nixal_reprap4040_rampsBracket (Autodesk Fusion 360 design; units mm, degrees)
Autodesk Fusion 360 part; units mm, degrees
sketch "Sketch1" plane through (0, 0, 0) normal (0, 1, 0) x (1, 0, 0)
  line L0 (0, 0) -> (135, 0)
  line L1 (135, 0) -> (135, 60)
  line L2 (135, 60) -> (0, 60)
  line L3 (0, 60) -> (0, 0)
  circle A0 centre (30, 10) radius 4
  circle A1 centre (105, 10) radius 4
  circle A2 centre (30, 50) radius 4
  circle A3 centre (105, 50) radius 4
  circle A4 centre (30, 10) radius 7.5
  circle A5 centre (105, 10) radius 7.5
  circle A6 centre (30, 50) radius 7.5
  circle A7 centre (105, 50) radius 7.5
  line L4 (0, 30) -> (135, 30) construction
  dimension "d1" = 135
  dimension "d2" = 60
  dimension "d3" = 8
  dimension "d4" = 8
  dimension "d5" = 10
  dimension "d6" = 10
  dimension "d7" = 75
  dimension "d8" = 30
  dimension "d9" = 20
  dimension "d10" = 8
  dimension "d11" = 8
  dimension "d12" = 10
  dimension "d13" = 10
  dimension "d14" = 15
  dimension "d15" = 15
  dimension "d16" = 15
  dimension "d17" = 15
  dimension "d18" = 30
  constraint horizontal L0
  constraint vertical L1
  constraint horizontal L2
  constraint vertical L3
  constraint coincident L0.start L3.end
  constraint concentric A0 A4
  constraint concentric A1 A5
  constraint concentric A2 A6
  constraint concentric A3 A7
  constraint coincident L3 L0.start
  constraint perpendicular L3 L4
  measures "d3" diameter of A0
  measures "d4" diameter of A1
  measures "d10" diameter of A2
  measures "d11" diameter of A3
  measures "d14" diameter of A4
  measures "d15" diameter of A5
  measures "d16" diameter of A6
  measures "d17" diameter of A7
  measures "d18" distance of L0 L4
extrude "Extrude1" add sketch "Sketch1" along normal blind 4 contours L0 L1 L2 L3 | A4 | A5 | A6 | A7 makes body 1
extrude "Extrude2" add sketch "Sketch1" along normal blind 6 separate body contours A4 | A5 makes body 2 at (112.4907, 4, -9.6262) makes body 3 at (37.4907, 4, -9.6262)
